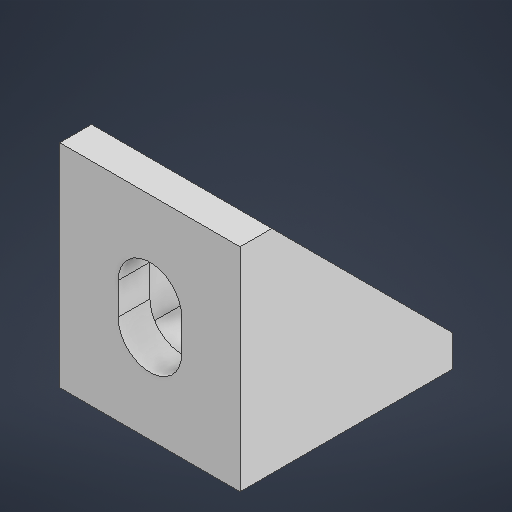
# Autodesk Inventor part: ANGULOESQUINA
Saved by Autodesk Inventor 2026.2 (Build 302298010, 298A)
## iProperties
Created: 2026-04-14
Part Number: ANGULOESQUINA
Material: Generic
Document SubType Name: Modeling
Designer: grego
Density: 1 g/cm^3
Appearance: Default
Author: grego
Autodesk Inventor part; units mm, degrees
ref_plane "YZ Plane" through (0, 0, 0) normal (1, 0, 0) x (0, 1, 0)
ref_plane "XZ Plane" through (0, 0, 0) normal (0, 1, 0) x (-1, 0, 0)
ref_plane "XY Plane" through (0, 0, 0) normal (0, 0, 1) x (1, 0, 0)
sketch "Sketch1" plane through (0, 0, 0) normal (0, 1, 0) x (-1, 0, 0)
  line L0 (0, 0) -> (-17, 0)
  line L1 (-17, 0) -> (-17, -20)
  line L2 (-17, -20) -> (0, -20)
  line L3 (0, -20) -> (0, 0)
  dimension "d0" = 17
  dimension "d1" = 20
  constraints: 8 end point, 2 parallel, 1 horizontal, 1 perpendicular
  measures "d0" distance of L2.end L1.end
  measures "d1" distance of L1.end L0.end
extrude "Extrusion1" add sketch "Sketch1" along normal blind 3
sketch "Sketch2" plane through (0, 3, 0) normal (0, 1, 0) x (1, 0, 0)
  line L0 (17, 0) -> (17, 20) projected
  line L1 (17, 20) -> (0, 20) projected
  line L2 (0, 20) -> (0, 0) projected
  line L3 (0, 0) -> (17, 0) projected
  line L4 (8.5, 14.5) -> (8.5, 14.5)
  line L5 (5.5, 11.5) -> (5.5, 8.5)
  line L6 (8.5, 5.5) -> (8.5, 5.5)
  line L7 (11.5, 8.5) -> (11.5, 11.5)
  arc A0 (8.5, 14.5) -> (5.5, 11.5) centre (8.5, 11.5) ccw
  arc A1 (11.5, 11.5) -> (8.5, 14.5) centre (8.5, 11.5) ccw
  arc A2 (5.5, 8.5) -> (8.5, 5.5) centre (8.5, 8.5) ccw
  arc A3 (8.5, 5.5) -> (11.5, 8.5) centre (8.5, 8.5) ccw
  point P0 (5.5, 5.5)
  point P1 (5.5, 14.5)
  point P2 (11.5, 5.5)
  dimension "d6" = 6
  dimension "d7" = 9
  dimension "d8" = 3
  constraints: 8 end point, 8 point on circle, 8 tangent, 6 point on line, 4 centre point, 3 equal radius, 2 parallel, 1 horizontal, 1 perpendicular
  measures "d6" distance of point (11.5, 5.5) point (5.5, 5.5)
  measures "d7" distance of point (5.5, 5.5) point (5.5, 14.5)
  measures "d8" radius of A0
extrude "Extrusion2" cut sketch "Sketch2" against normal blind 3 contours A0 A1 L7 A3 A2 L5
sketch "Sketch3" plane through (0, 3, 0) normal (0, 1, 0) x (1, 0, 0)
  line L0 (11.5, 11.5) -> (11.5, 8.5) projected
  arc A0 (5.5, 8.5) -> (11.5, 8.5) centre (8.5, 8.5) ccw projected
  line L1 (5.5, 8.5) -> (5.5, 11.5) projected
  arc A1 (11.5, 11.5) -> (5.5, 11.5) centre (8.5, 11.5) ccw projected
  line L2 (17, 0) -> (17, 20) projected
  line L3 (17, 20) -> (0, 20) projected
  line L4 (0, 20) -> (0, 0) projected
  line L5 (0, 0) -> (17, 0) projected
  line L6 (0, 20) -> (0, 0) projected
  line L7 (0, 0) -> (17, 0)
  line L8 (17, 0) -> (17, 3)
  line L9 (17, 3) -> (0, 3)
  line L10 (0, 3) -> (0, 0)
  dimension "d11" = 3
  constraints: 8 end point, 2 parallel, 1 horizontal, 1 perpendicular, 1 point on line
  measures "d11" distance of L8.end L7.end
extrude "Extrusion3" add sketch "Sketch3" along normal blind 17 contours L5 L4 L9 L2
sketch "Sketch4" plane through (0, 0, 0) normal (0, 0, 1) x (1, 0, 0)
  line L0 (0, 0) -> (17, 0) projected
  line L1 (17, 0) -> (17, 20) projected
  line L2 (0, 20) -> (17, 20) projected
  line L3 (0, 0) -> (0, 20) projected
  line L4 (8.5, 5.5) -> (8.5, 5.5)
  line L5 (11.5, 8.5) -> (11.5, 11.5)
  line L6 (8.5, 14.5) -> (8.5, 14.5)
  line L7 (5.5, 11.5) -> (5.5, 8.5)
  line L8 (5.5, 5.5) -> (11.5, 14.5) construction
  line L9 (11.5, 5.5) -> (5.5, 14.5) construction
  arc A0 (8.5, 14.5) -> (5.5, 11.5) centre (8.5, 11.5) ccw
  arc A1 (11.5, 11.5) -> (8.5, 14.5) centre (8.5, 11.5) ccw
  arc A2 (5.5, 8.5) -> (8.5, 5.5) centre (8.5, 8.5) ccw
  arc A3 (8.5, 5.5) -> (11.5, 8.5) centre (8.5, 8.5) ccw
  point P0 (8.5, 10)
  dimension "d14" = 6
  dimension "d15" = 9
  dimension "d16" = 3
  constraints: 12 end point, 8 point on circle, 8 point on line, 8 tangent, 4 centre point, 3 equal radius, 2 midpoint, 2 parallel, 1 horizontal, 1 perpendicular
  measures "d14" distance of L9.end L8.end
  measures "d15" distance of L8.end L9.start
  measures "d16" radius of A0
extrude "Extrusion4" cut sketch "Sketch4" against normal blind 3 contours A3 A2 L7 A0 A1 L5
sketch "Sketch5" plane through (17, 0, 0) normal (1, 0, 0) x (0, 0, -1)
  line L0 (0, 0) -> (20, 0) projected
  line L1 (20, 0) -> (20, 3) projected
  line L2 (3, 3) -> (20, 3) projected
  line L3 (3, 3) -> (3, 20) projected
  line L4 (0, 20) -> (3, 20) projected
  line L5 (0, 0) -> (0, 20) projected
  line L6 (20, 3) -> (3, 20)
  constraints: 2 end point
extrude "Extrusion5" add sketch "Sketch5" against normal blind 2 contours L2 L3 L6
sketch "Sketch6" plane through (0, 0, -20) normal (-1, 0, 0) x (0, 0, 1)
  line L0 (17, 3) -> (0, 3) projected
  line L1 (17, 3) -> (17, 20) projected
  line L2 (0, 3) -> (17, 20)
  line L3 (0, 0) -> (20, 0) projected
  line L4 (20, 0) -> (20, 20) projected
  line L5 (17, 20) -> (20, 20) projected
  line L6 (17, 3) -> (17, 20) projected
  line L7 (0, 3) -> (17, 3) projected
  line L8 (0, 0) -> (0, 3) projected
  constraints: 2 end point
extrude "Extrusion6" add sketch "Sketch6" against normal blind 2 contours L0 L2 L1
body "Solid1"
